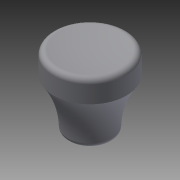
# Autodesk Inventor part: pushbutton
Saved by Autodesk Inventor 2013 (Build 170138000, 138)
## iProperties
Created: 2013-01-11
Part Number: pushbutton
Material: Generic
Document SubType Name: Modeling
Designer: md
Density: 1 g/cm^3
Author: md
Autodesk Inventor part; units mm, degrees
ref_plane "YZ Plane" through (0, 0, 0) normal (1, 0, 0) x (0, 1, 0)
ref_plane "XZ Plane" through (0, 0, 0) normal (0, 1, 0) x (-1, 0, 0)
ref_plane "XY Plane" through (0, 0, 0) normal (0, 0, 1) x (1, 0, 0)
sketch "Sketch1" plane through (0, 0, 0) normal (0, 1, 0) x (-1, 0, 0)
  line L0 (1.6, 0) -> (1.6, 10)
  line L1 (1.6, 10) -> (0, 10)
  line L2 (0, 10) -> (0, 13.9674)
  line L3 (7.5, 14.7071) -> (7.5, 10)
  line L4 (4.55, 0) -> (1.6, 0)
  arc A0 (0, 13.9674) -> (7.5, 14.7071) centre (0.1821, 50.5137) ccw
  arc A1 (7.5, 10) -> (4.55, 0) centre (20.9678, 0.5919) ccw
  point P0 (0, 0)
  dimension "d0" = 1.6
  dimension "d5" = 10
  dimension "d9" = 7.5
  dimension "d10" = 0
  dimension "d11" = 36.5468
  dimension "d12" = 3.9674
  dimension "d13" = 5.9
  dimension "d16" = 14.7071
  dimension "d17" = 16.4285
  dimension "d18" = 2.95
  dimension "d20" = 20.9678
  constraints: 10 end point, 4 point on circle, 3 parallel, 2 centre point, 1 perpendicular, 1 vertical
  measures "d0" distance of L0.end L1.end
  measures "d5" distance of L0.start L0.end
  measures "d9" distance from line of point (0, 0) L3
  measures "d10" distance from line of point (0, 0) L4
  measures "d11" radius of A0
  measures "d12" distance of L1.end L2.end
  measures "d13" distance between parallel lines of L0 L3
  measures "d16" distance from line of L3.start L4
  measures "d17" radius of A1
  measures "d18" distance of L4.start L0.start
  measures "d20" horizontal distance of A1.centre point (0, 0)
revolve "Revolution1" add sketch "Sketch1" angle 360 about axis through (0, 0, 10) along (0, 0, 1)
fillet "Fillet1" radius 1 2 edges at (4.55, 0, 0) (7.5, 0, 14.7071)
equation "\"d0\" = 0.5 * LSH_Durchmesser + epsilon"
equation "\"d9\" = 0.5 * Taster_Durchmesser"
equation "\"d15\" = Rundung"
equation "\"LSH_Durchmesser\" = 3"
equation "\"epsilon\" = 0.1"
equation "\"Taster_Durchmesser\" = 15"
equation "\"Rundung\" = 1"
body "Solid1"
